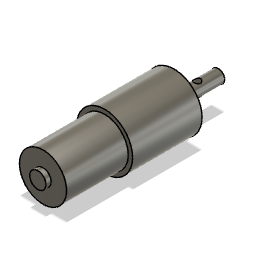
motorreductor v4 (Autodesk Fusion 360 design; units mm, degrees)
Autodesk Fusion 360 part; units mm, degrees
note: some values were not read from the file. Set by a fixed rule: which sketch regions a step uses.
sketch "Boceto1" plane through (0, 0, 0) normal (0, 0, 1) x (1, 0, 0)
  circle A0 centre (0, 0) radius 14.45
  circle A1 centre (0, 0) radius 17.125
  circle A2 centre (0, 0) radius 4
  circle A3 centre (0, 0) radius 5
  circle A4 centre (0, 0) radius 8
  line L0 (0, 0) -> (0, 11.225)
  circle A5 centre (0, 11.225) radius 1.5
  circle A6 centre (-11.225, 0) radius 1.5
  circle A7 centre (0, -11.225) radius 1.5
  circle A8 centre (11.225, 0) radius 1.5
  dimension "d1" = 28.9
  dimension "d2" = 34.25
  dimension "d7" = 8
  dimension "d8" = 10
  dimension "d13" = 16
  dimension "d22" = 11.225
  dimension "d23" = 3
  dimension "d25" = 360
  constraint coincident A0.centre A1.centre
  constraint concentric A0 A1
  constraint concentric A0 A2
  constraint concentric A2 A3
  constraint vertical L0
  constraint coincident L0.end A5.centre
  measures "d1" diameter of A0
  measures "d2" diameter of A1
  measures "d7" diameter of A2
  measures "d8" diameter of A3
  measures "d13" diameter of A4
  measures "d22" distance of A0.centre L0.end
  measures "d23" diameter of A5
extrude "Extruir1" add sketch "Boceto1" along normal blind 80.4 contours A0 | A2 | A3 | A4 | A5 | A6 | A7 | A8
extrude "Extruir2" add sketch "Boceto1" along normal blind 42.6 contours A1
extrude "Extruir3" add sketch "Boceto1" along normal blind 83.6 contours A2 | A3
extrude "Extruir4" add sketch "Boceto1" against normal blind 27 contours A2
extrude "Extruir5" add sketch "Boceto1" against normal blind 1.7 contours A4
sketch "Boceto2" plane through (0, 0, 0) normal (0, 1, 0) x (1, 0, 0)
  line L0 (4, 27) -> (4, 2.5)
  line L1 (-4, 2.5) -> (-4, 27)
  line L2 (4, 27) -> (-4, 27)
  line L3 (4, 27) -> (-4, 27)
  line L4 (-4, 0) -> (4, 0)
  line L5 (4, 27) -> (-4, 27)
  line L6 (0, 27) -> (0, 16.1)
  line L7 (0, 16.1) -> (0, 14.1)
  circle A0 centre (0, 14.1) radius 2
  dimension "d26" = 10.9
  dimension "d27" = 2
  dimension "d28" = 4
  constraint vertical L0
  constraint vertical L1
  constraint midpoint L2 L6.start
  constraint perpendicular L2 L6
  constraint parallel L6 L7
  constraint coincident L7.end A0.centre
  measures "d26" distance of L6.start L6.end
  measures "d27" distance of L6.end L7.end
  measures "d28" diameter of A0
extrude "Extruir7" cut sketch "Boceto2" along normal mid plane 14
